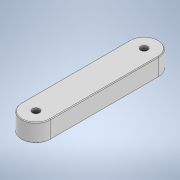
# Autodesk Inventor part: Link2_3
Saved by Autodesk Inventor 2022 (Build 260153000, 153)
## iProperties
Created: 2022-01-31
Part Number: Link2_3
Material: Generic
Document SubType Name: Modeling
Designer: Leonardo
Density: 1 g/cm^3
Appearance: Default
Author: Leonardo
Autodesk Inventor part; units mm, degrees
ref_plane "YZ Plane" through (0, 0, 0) normal (1, 0, 0) x (0, 1, 0)
ref_plane "XZ Plane" through (0, 0, 0) normal (0, 1, 0) x (-1, 0, 0)
ref_plane "XY Plane" through (0, 0, 0) normal (0, 0, 1) x (1, 0, 0)
sketch "Sketch1" plane through (0, 0, 0) normal (0, 1, 0) x (-1, 0, 0)
  circle A0 centre (0, 0) radius 40
  circle A1 centre (0, 0) radius 10
  circle A2 centre (0, -300) radius 40
  circle A3 centre (0, -300) radius 10
  line L0 (40, 0) -> (40, -300)
  line L1 (-40, 0) -> (-40, -300)
  dimension "d0" = 80
  dimension "d1" = 20
  dimension "d2" = 80
  dimension "d3" = 20
  dimension "d4" = 300
  constraints: 4 centre point, 4 end point, 4 point on circle, 3 coincident, 2 tangent, 1 parallel, 1 vertical
  measures "d0" diameter of A0
  measures "d1" diameter of A1
  measures "d2" diameter of A2
  measures "d3" diameter of A3
  measures "d4" distance of L0.start L0.end
extrude "Extrusion1" add sketch "Sketch1" along normal blind 50
fillet "Fillet1" radius 2 8 edges at (0, 50, -340) (-40, 50, -150) (0, 50, 40) (40, 50, -150) (0, 0, -340) (-40, 0, -150) (0, 0, 40) (40, 0, -150)
body "Solid1"
